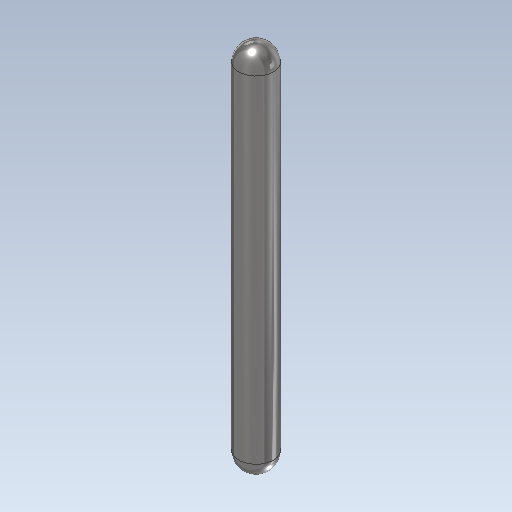
# Autodesk Inventor part: 99a-1047031000
Saved by Autodesk Inventor 2020 (Build 240168000, 168)
## iProperties
Created: 2013-01-10
Part Number: 99a-1047031000
Material: Stainless Steel
Document SubType Name: Modeling
Designer: Mark Neilson
Mass: 0.0130562 g
Surface Area: 0.114212 cm^2
Volume: 0.00161587 cm^3
Density: 8.08 g/cm^3
Appearance: Semi-Polished
Description: Mini BTE Cross Pin
Company: InTech
Author: Mark Neilson
Autodesk Inventor part; units mm, degrees
ref_plane "YZ Plane" through (0, 0, 0) normal (1, 0, 0) x (0, 1, 0)
ref_plane "XZ Plane" through (0, 0, 0) normal (0, 1, 0) x (-1, 0, 0)
ref_plane "XY Plane" through (0, 0, 0) normal (0, 0, 1) x (1, 0, 0)
sketch "Sketch1-<F>" plane through (0, 0, 0) normal (0, 0, 1) x (1, 0, 0)
  circle A0 centre (0, 0) radius 0.2921
  dimension "d3" = 0.5842
  constraints: 1 centre point, 1 other
  measures "d3" diameter of A0
extrude "Midplane_HP" add sketch "Sketch1-<F>" along normal mid plane 6.223
fillet "Fillet2" radius 0.2921 2 edges at (-0.2921, 0, 3.1115) (-0.2921, 0, -3.1115)
equation "\"mdt_d0\" = 0"
equation "\"mdt_d3\" = 0.011"
body "Solid1"
